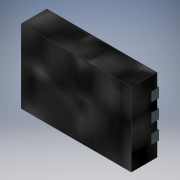
# Autodesk Inventor part: DFN-6-1EP_3x2mm_P0.5mm_EP1.65x1.35mm
Saved by Autodesk Inventor 2019.1 (Build 231200000, 200)
## iProperties
Created: 2018-11-01
Part Number: DFN-6-1EP_3x2mm_P0.5mm_EP1.65x1.35mm
Material: Generic
Document SubType Name: Modeling
Designer: huesof
Density: 1 g/cm^3
Appearance: Default
Author: huesof
Autodesk Inventor part; units mm, degrees
sketch "Sketch1" plane through (0, 0, 0) normal (0, 0, 1) x (1, 0, 0)
  line L0 (-1.5, -1) -> (1.5, -1)
  line L1 (1.5, -1) -> (1.5, 1)
  line L2 (1.5, 1) -> (-1.5, 1)
  line L3 (-1.5, 1) -> (-1.5, -1)
  line L4 (-1.5, -1) -> (1.5, 1) construction
  line L5 (1.5, -1) -> (-1.5, 1) construction
  line L6 (-1.5, 0.375) -> (-1.215, 0.375)
  line L7 (-1.1, 0.49) -> (-1.1, 0.51)
  line L8 (-1.215, 0.625) -> (-1.5, 0.625)
  line L9 (-1.5, 0.625) -> (-1.5, 0.375)
  line L10 (-1.5, 0.375) -> (-1.1, 0.625) construction
  line L11 (-1.1, 0.375) -> (-1.5, 0.625) construction
  arc A0 (-1.215, 0.375) -> (-1.1, 0.49) centre (-1.215, 0.49) ccw
  arc A1 (-1.1, 0.51) -> (-1.215, 0.625) centre (-1.215, 0.51) ccw
  line L12 (0, 1) -> (0, -1) construction
  line L13 (1.5, 0.375) -> (1.215, 0.375)
  line L14 (1.1, 0.49) -> (1.1, 0.51)
  line L15 (1.215, 0.625) -> (1.5, 0.625)
  line L16 (1.5, 0.625) -> (1.5, 0.375)
  arc A2 (1.1, 0.49) -> (1.215, 0.375) centre (1.215, 0.49) ccw
  arc A3 (1.215, 0.625) -> (1.1, 0.51) centre (1.215, 0.51) ccw
  line L17 (-1.5, 0.125) -> (-1.5, -0.125)
  line L18 (-1.215, 0.125) -> (-1.5, 0.125)
  arc A4 (-1.1, 0.01) -> (-1.215, 0.125) centre (-1.215, 0.01) ccw
  arc A5 (-1.215, -0.125) -> (-1.1, -0.01) centre (-1.215, -0.01) ccw
  line L19 (-1.1, -0.01) -> (-1.1, 0.01)
  line L20 (-1.5, -0.125) -> (-1.215, -0.125)
  line L21 (1.5, 0.125) -> (1.5, -0.125)
  line L22 (1.5, -0.125) -> (1.215, -0.125)
  line L23 (1.215, 0.125) -> (1.5, 0.125)
  arc A6 (1.1, -0.01) -> (1.215, -0.125) centre (1.215, -0.01) ccw
  line L24 (1.1, -0.01) -> (1.1, 0.01)
  arc A7 (1.215, 0.125) -> (1.1, 0.01) centre (1.215, 0.01) ccw
  line L25 (-1.5, -0.375) -> (-1.5, -0.625)
  line L26 (-1.215, -0.375) -> (-1.5, -0.375)
  arc A8 (-1.1, -0.49) -> (-1.215, -0.375) centre (-1.215, -0.49) ccw
  arc A9 (-1.215, -0.625) -> (-1.1, -0.51) centre (-1.215, -0.51) ccw
  line L27 (-1.1, -0.51) -> (-1.1, -0.49)
  line L28 (-1.5, -0.625) -> (-1.215, -0.625)
  line L29 (1.5, -0.375) -> (1.5, -0.625)
  line L30 (1.5, -0.625) -> (1.215, -0.625)
  line L31 (1.215, -0.375) -> (1.5, -0.375)
  arc A10 (1.1, -0.51) -> (1.215, -0.625) centre (1.215, -0.51) ccw
  line L32 (1.1, -0.51) -> (1.1, -0.49)
  arc A11 (1.215, -0.375) -> (1.1, -0.49) centre (1.215, -0.49) ccw
  line L33 (-0.825, -0.675) -> (0.825, -0.675)
  line L34 (0.825, -0.675) -> (0.825, 0.675)
  line L35 (0.825, 0.675) -> (-0.625, 0.675)
  line L36 (-0.825, 0.675) -> (-0.825, -0.675) construction
  line L37 (-0.825, -0.675) -> (0.825, 0.675) construction
  line L38 (0.825, -0.675) -> (-0.825, 0.675) construction
  arc A12 (-0.825, 0.475) -> (-0.625, 0.675) centre (-0.825, 0.675) ccw
  line L39 (-0.825, 0.675) -> (-0.825, 0.55) construction
  line L40 (-0.825, 0.675) -> (-0.625, 0.675) construction
  line L41 (-0.625, 0.675) -> (-0.825, 0.675) construction
  line L42 (-0.825, 0.55) -> (-0.825, 0.475) construction
  line L43 (-0.825, -0.675) -> (-0.825, 0.475)
  point P0 (0, 0)
  point P1 (-1.3, 0.5)
  point P2 (-1.1, 0.125)
  point P3 (-1.1, -0.125)
  point P4 (-1.1, -0.375)
  point P5 (-1.1, -0.625)
  dimension "d0" = 3
  dimension "d1" = 2
  dimension "d2" = 0.4
  dimension "d3" = 0.25
  dimension "d4" = 0.5
  dimension "d5" = 0.115
  dimension "d8" = 0.5
  dimension "d32" = 1.65
  dimension "d33" = 1.35
  dimension "d34" = 0.2
  dimension "d35" = 90
  constraints: 88 end point, 26 point on circle, 13 centre point, 13 point on line, 8 midpoint, 8 symmetric about line, 7 parallel, 4 tangent, 3 collinear, 3 horizontal, 3 perpendicular, 1 coincident, 1 equal radius, 1 vertical, 61 other
  measures "d0" distance of L2.end L1.end
  measures "d1" distance of L1.end L0.end
  measures "d2" distance of L8.end L10.end
  measures "d3" distance of L10.end L11.start
  measures "d4" vertical distance of point (0, 0) point (-1.3, 0.5)
  measures "d5" radius of A0
  measures "d8" distance of L8.end L17.start
  measures "d32" distance of L36.start L34.end
  measures "d33" distance of L34.end L33.end
  measures "d34" radius of A12
  measures "d35" angle of L39 L40
ref_plane "Work Plane1" through (0, 0, 0.75) normal (0, 0, 1) x (1, 0, 0)
ref_plane "Work Plane2" through (0, 0, 0.05) normal (0, 0, 1) x (1, 0, 0)
ref_plane "Work Plane3" through (0, 0, 0.2) normal (0, 0, 1) x (1, 0, 0)
extrude "Extrusion2" add sketch "Sketch1" along normal up to surface (0.55 mm away) from surface at 0.2 contours L3 L28 A9 L27 A8 L26 L20 A5 L19 A4 L18 L6 A0 L7 A1 L8 L2 L1 L15 A3 L14 A2 L13 L23 A7 L24 A6 L22 L31 A11 L32 A10 L30 L0 | L3 L26 A8 L27 A9 L28 | L30 A10 L32 A11 L31 L1 | L3 L18 A4 L19 A5 L20 | L22 A6 L24 A7 L23 L1 | L3 L8 A1 L7 A0 L6 | L13 A2 L14 A3 L15 L1 | L43 A12 L35 L34 L33
extrude "Extrusion3" add sketch "Sketch1" along normal up to surface (0.15 mm away) from surface at 0.05 contours L3 L28 A9 L27 A8 L26 L20 A5 L19 A4 L18 L6 A0 L7 A1 L8 L2 L1 L15 A3 L14 A2 L13 L23 A7 L24 A6 L22 L31 A11 L32 A10 L30 L0
extrude "Extrusion4" add sketch "Sketch1" along normal up to surface (0.2 mm away) from surface at 0 separate body contours L3 L26 A8 L27 A9 L28 | L30 A10 L32 A11 L31 L1 | L3 L18 A4 L19 A5 L20 | L22 A6 L24 A7 L23 L1 | L3 L8 A1 L7 A0 L6 | L13 A2 L14 A3 L15 L1 | L43 A12 L35 L34 L33
body "Solid2"
body "Solid3"
